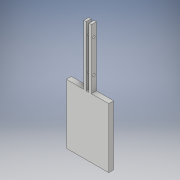
# Autodesk Inventor part: 2BarClawPaddle
Saved by Autodesk Inventor 2017 (Build 210142000, 142)
## iProperties
Created: 2017-09-30
Part Number: 2BarClawPaddle
Material: Generic
Document SubType Name: Modeling
Designer: User
Density: 1 g/cm^3
Appearance: Default
Author: User
Autodesk Inventor part; units mm, degrees
ref_plane "YZ Plane" through (0, 0, 0) normal (1, 0, 0) x (0, 1, 0)
ref_plane "XZ Plane" through (0, 0, 0) normal (0, 1, 0) x (-1, 0, 0)
ref_plane "XY Plane" through (0, 0, 0) normal (0, 0, 1) x (1, 0, 0)
sketch "Sketch1" plane through (0, 0, 0) normal (0, 0, 1) x (1, 0, 0)
  line L0 (0, 0) -> (53.975, 0)
  line L1 (0, 0) -> (0, -76.2)
  line L2 (0, -76.2) -> (53.975, -76.2)
  line L3 (53.975, -76.2) -> (53.975, 0)
  dimension "d1" = 53.975
  dimension "d2" = 76.2
  dimension "d3" = 53.975
  constraints: 8 end point, 1 horizontal, 1 perpendicular, 1 vertical
  measures "d1" distance of L0.start L0.end
  measures "d2" distance of L0.start L1.end
  measures "d3" distance of L1.end L2.end
extrude "Extrusion1" add sketch "Sketch1" along normal blind 3.175
sketch "Sketch2" plane through (0, 0, 0) normal (0, 1, 0) x (1, 0, 0)
  line L0 (53.975, -3.175) -> (0, -3.175) projected
  line L1 (25.3873, -1.5875) -> (25.3873, 0)
  line L2 (25.3873, -3.175) -> (25.3873, -1.5875)
  line L3 (28.7401, -1.5875) -> (28.7401, -3.175)
  line L4 (28.7401, -1.5875) -> (28.7401, 0)
  line L5 (25.3873, -3.175) -> (22.2123, -3.175)
  line L6 (22.2123, -3.175) -> (22.2123, 3.175)
  line L7 (28.7401, -3.175) -> (31.9151, -3.175)
  line L8 (31.9151, -3.175) -> (31.9151, 3.175)
  line L9 (25.3873, 0) -> (25.3873, 3.175)
  line L10 (25.3873, 3.175) -> (22.2123, 3.175)
  line L11 (31.9151, 3.175) -> (28.7401, 3.175)
  line L12 (28.7401, 3.175) -> (28.7401, 0)
  point P0 (27.0637, -1.5875)
  dimension "d7" = 1.6764
  dimension "d8" = 1.6764
  dimension "d9" = 3.175
  dimension "d10" = 6.35
  dimension "d11" = 3.175
  constraints: 24 end point, 7 point on line, 4 perpendicular, 1 collinear, 1 vertical
  measures "d7" distance of point (27.064, -1.587) L3.start
  measures "d8" distance of point (27.064, -1.587) L1.start
  measures "d9" distance of L2.start L5.end
  measures "d10" distance of L5.end L6.end
  measures "d11" distance of L3.end L7.end
sketch "Sketch3" plane through (0, 0, 0) normal (0, 0, -1) x (-1, 0, 0)
  line L0 (-53.975, 0) -> (0, 0) projected
  line L1 (0, -76.2) -> (-53.975, -76.2) projected
  line L2 (0, 0) -> (-53.975, 0)
  line L3 (-53.975, 0) -> (-53.975, -76.2)
  line L4 (-53.975, -76.2) -> (0, -76.2)
  line L5 (0, -76.2) -> (0, 0)
  constraints: 8 end point, 2 parallel, 1 horizontal, 1 perpendicular
extrude "Extrusion2" add sketch "Sketch3" along normal blind 3.175
extrude "Extrusion3" add sketch "Sketch2" along normal blind 76.2 contours L0 L3 L4 L12 L11 L8
extrude "Extrusion4" add sketch "Sketch2" along normal blind 76.2 contours L0 L6 L10 L9 L1 L2
sketch "Sketch4" plane through (31.9151, 0, 3.175) normal (1, 0, 0) x (0, 0, -1)
  line L0 (3.175, 0) -> (3.175, 19.05)
  circle A0 centre (3.175, 19.05) radius 1.5875
  dimension "d18" = 19.05
  dimension "d19" = 3.175
  constraints: 2 end point, 1 centre point, 1 coincident, 1 vertical
  measures "d18" distance of L0.start L0.end
  measures "d19" diameter of A0
extrude "Extrusion5" cut sketch "Sketch4" against normal blind 50.8
sketch "Sketch5" plane through (31.9151, 0, 3.175) normal (1, 0, 0) x (0, 0, -1)
  circle A0 centre (3.175, 19.05) radius 1.5875 projected
  line L0 (3.175, 19.05) -> (3.175, 60.706)
  circle A1 centre (3.175, 60.706) radius 1.5875
  point P0 (3.175, 0)
  dimension "d22" = 41.656
  dimension "d23" = 3.175
  constraints: 2 end point, 1 centre point, 1 coincident, 1 vertical
  measures "d22" distance of L0.start L0.end
  measures "d23" diameter of A1
extrude "Extrusion6" cut sketch "Sketch5" against normal blind 50.8 contours A1
body "Solid1"
